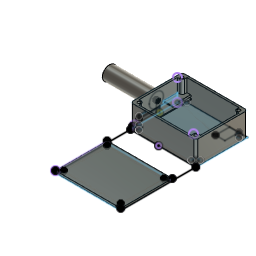
modelo para la plaqueta del nivel v13 (Autodesk Fusion 360 design; units mm, degrees)
Autodesk Fusion 360 part; units mm, degrees
sketch "Boceto1" plane through (0, 0, 0) normal (0, 0, 1) x (1, 0, 0)
  line L0 (39.56, 0) -> (39.56, 55)
  line L1 (39.56, 55) -> (-30, 55)
  line L2 (-30, 55) -> (-30, 0)
  line L3 (-30, 0) -> (39.56, 0)
  dimension "d136" = 55
  dimension "d137" = 69.56
  constraint vertical L0
  constraint horizontal L1
  constraint perpendicular L1 L2
  constraint parallel L1 L3
  constraint coincident origin L3
  measures "d136" distance of L1.end L2.end
  measures "d137" distance of L0.end L1.end
extrude "Extruir1" add sketch "Boceto1" along normal blind 25 makes body 1
shell "Vaciado1" thickness 2 removed faces 1 at (16.3733, 18.3333, 25) on bodies 1
sketch "Boceto2" plane through (0, 0, 0) normal (0, 0, 1) x (1, 0, 0)
  line L0 (-30, -25) -> (39.56, -25)
  line L1 (39.56, -25) -> (39.56, -80)
  line L2 (39.56, -80) -> (-30, -80)
  line L3 (-30, -25) -> (-30, -80)
  line L4 (-30, 0) -> (-30, -25)
  line L5 (39.56, 0) -> (39.56, -25)
  point P0 (-30, 0)
  point P1 (39.56, 0)
  constraint horizontal L0
  constraint vertical L1
  constraint horizontal L2
  constraint perpendicular L2 L3
  constraint coincident P0 L4.start
  constraint perpendicular L0 L4
  constraint coincident P1 L5.start
  constraint perpendicular L0 L5
extrude "Extruir2" add sketch "Boceto2" along normal blind 2 separate body makes body 2
sketch "Boceto7" plane through (0, 0, 2) normal (0, 0, 1) x (-1, 0, 0)
  line L0 (28, -2) -> (-37.56, -2)
  line L1 (-37.56, -2) -> (-37.56, -53)
  line L2 (-37.56, -53) -> (28, -53)
  line L3 (28, -53) -> (28, -2)
  circle A0 centre (25.5, -50.5) radius 2.5
  circle A1 centre (25.5, -4.5) radius 2.5
  circle A2 centre (-35.06, -4.5) radius 2.5
  circle A3 centre (-35.06, -50.5) radius 2.5
  line L4 (23, -50.5) -> (23, -53)
  line L5 (28, -47.9255) -> (25.4266, -48.0011)
  line L6 (25.5, -7) -> (28, -7)
  line L7 (23, -4.5) -> (23, -2)
  line L8 (-32.56, -4.5) -> (-32.56, -2)
  line L9 (-35.06, -7) -> (-37.56, -7)
  line L10 (-34.9754, -48.0014) -> (-37.56, -47.9139)
  line L11 (-32.5302, -53) -> (-32.5602, -50.4704)
  dimension "d26" = 5
  dimension "d27" = 5
  dimension "d28" = 5
  dimension "d29" = 5
  constraint tangent L2 A0
  constraint tangent L3 A0
  constraint tangent L0 A1
  constraint tangent L3 A1
  constraint tangent L1 A3
  constraint tangent L1 A2
  constraint tangent L2 A3
  constraint tangent L0 A2
  constraint coincident A0 L4.start
  constraint coincident L2 L4.end
  constraint tangent A0 L4
  constraint coincident A0 L5.end
  constraint coincident L3 L5.start
  constraint tangent A0 L5
  constraint coincident A1 L6.start
  constraint coincident L3 L6.end
  constraint tangent A1 L6
  constraint coincident A1 L7.start
  constraint coincident L0 L7.end
  constraint tangent A1 L7
  constraint coincident A2 L8.start
  constraint coincident L0 L8.end
  constraint perpendicular L0 L8
  constraint coincident A2 L9.start
  constraint coincident L1 L9.end
  constraint tangent A2 L9
  constraint coincident A3 L10.start
  constraint coincident L1 L10.end
  constraint tangent A3 L10
  constraint coincident A3 L11.end
  constraint coincident L2 L11.start
  constraint tangent A3 L11
  measures "d26" diameter of A0
  measures "d27" diameter of A1
  measures "d28" diameter of A2
  measures "d29" diameter of A3
extrude "Extruir4" add sketch "Boceto7" along normal blind 23 separate body contours A1 | A2 | A0 | A3 L11 makes body 3 at (-27.9876, 50.2511, 17.3333) makes body 4 at (32.5631, 50.6246, 9.6667) makes body 5 at (-27.9969, 4.6246, 9.6667) makes body 6 at (35.7371, 6.9066, 17.3333)
extrude "Extruir5" add sketch "Boceto7" along normal blind 23 contours L0 A1 L7 | L0 A2 L8 | L0 L3 A1 | L0 L1 A2 | L3 A1 L6 | L1 A2 L9 | L3 A0 L5 | L1 A3 L10 | L2 L3 A0 | L1 L2 A3 | L2 A0 L4 | L2 A3 L11 bodies 1 3 4 5 6
sketch "Boceto8" plane through (0, 0, 25) normal (0, 0, 1) x (-1, 0, 0)
  line L0 (30, 0) -> (-39.56, 0)
  line L1 (-39.56, 0) -> (-39.56, -55)
  line L2 (-39.56, -55) -> (30, -55)
  line L3 (30, -55) -> (30, 0)
  arc A0 (25.4266, -48.0011) -> (23, -50.5) centre (25.5, -50.5) ccw
  line L4 (23, -50.5) -> (23, -53)
  line L5 (23, -53) -> (-32.5302, -53)
  line L6 (-32.5302, -53) -> (-32.5602, -50.4704)
  arc A1 (-32.5602, -50.4704) -> (-34.9754, -48.0014) centre (-35.06, -50.5) ccw
  line L7 (-34.9754, -48.0014) -> (-37.56, -47.9139)
  line L8 (-37.56, -47.9139) -> (-37.56, -7)
  line L9 (-37.56, -7) -> (-35.06, -7)
  arc A2 (-35.06, -7) -> (-32.56, -4.5) centre (-35.06, -4.5) ccw
  line L10 (-32.56, -4.5) -> (-32.56, -2)
  line L11 (-32.56, -2) -> (23, -2)
  line L12 (23, -2) -> (23, -4.5)
  arc A3 (23, -4.5) -> (25.5, -7) centre (25.5, -4.5) ccw
  line L13 (25.5, -7) -> (28, -7)
  line L14 (28, -7) -> (28, -47.9255)
  line L15 (28, -47.9255) -> (25.4266, -48.0011)
chamfer "Chaflán4" distance 2 angle 45 1 edges at (39.56, 0, 12.5) on bodies 1
chamfer "Chaflán4" distance 2 angle 45 3 edges at (-30, 0, 12.5) (39.56, 55, 12.5) (-30, 55, 12.5) on bodies 1
chamfer "Chaflán5" distance 2 angle 45 4 edges at (-30, -80, 1) (39.56, -80, 1) (-30, -25, 1) (39.56, -25, 1) on bodies 2
hole "Agujero1" at (-25.5, 50.5, 25) direction (0, 0, -1) diameter 3 depth 20 tip angle 180 bodies 1
hole "Agujero2" at (-25.5, 4.5, 25) direction (0, 0, -1) diameter 3 depth 20 tip angle 180 bodies 1
hole "Agujero7" at (35.06, 4.5, 25) direction (0, 0, -1) diameter 3 depth 20 tip angle 180 bodies 1
hole "Agujero8" at (35.06, 50.5, 25) direction (0, 0, -1) diameter 3 depth 20 tip angle 180 bodies 1
sketch "Boceto9" plane through (0, 0, 2) normal (0, 0, 1) x (-1, 0, 0)
  line L0 (-39.56, 27) -> (-37.56, 25)
  line L1 (-37.56, 25) -> (28, 25)
  line L2 (28, 25) -> (30, 27)
  line L3 (30, 27) -> (30, 78)
  line L4 (30, 78) -> (28, 80)
  line L5 (28, 80) -> (-37.56, 80)
  line L6 (-37.56, 80) -> (-39.56, 78)
  line L7 (-39.56, 78) -> (-39.56, 27)
  circle A0 centre (25.5, 75.5) radius 1.5
  line L8 (30, 25) -> (30, 80)
  circle A1 centre (25.5, 29.5) radius 1.5
  circle A2 centre (-35.06, 75.5) radius 1.5
  circle A3 centre (-35.06, 29.5) radius 1.5
  line L9 (30, 25) -> (25.5, 25)
  line L10 (25.5, 25) -> (25.5, 29.5)
  line L11 (30, 80) -> (25.5, 80)
  line L12 (25.5, 80) -> (25.5, 75.5)
  line L13 (-39.56, 80) -> (-35.06, 80)
  line L14 (-35.06, 80) -> (-35.06, 75.5)
  line L15 (-39.56, 25) -> (-39.56, 29.5)
  line L16 (-39.56, 29.5) -> (-35.06, 29.5)
  point P0 (30, 80)
  point P1 (-39.56, 80)
  point P2 (-39.56, 25)
  dimension "d76" = 3
  dimension "d87" = 3
  dimension "d93" = 3
  dimension "d94" = 3
  dimension "d140" = 4.5
  dimension "d141" = 4.5
  dimension "d142" = 4.5
  dimension "d143" = 4.5
  dimension "d144" = 4.5
  dimension "d145" = 4.5
  dimension "d146" = 4.5
  dimension "d147" = 4.5
  constraint coincident L8.start L9.start
  constraint perpendicular L8 L9
  constraint perpendicular L1 L10
  constraint coincident A1.centre L10.end
  constraint coincident P0 L8.end
  constraint perpendicular L8 L11
  constraint perpendicular L11 L12
  constraint coincident A0.centre L12.end
  constraint coincident P1 L13.start
  constraint parallel L5 L13
  constraint perpendicular L5 L14
  constraint coincident A2.centre L14.end
  constraint coincident P2 L15.start
  constraint parallel L7 L15
  constraint perpendicular L7 L16
  constraint coincident A3.centre L16.end
  measures "d76" diameter of A0
  measures "d87" diameter of A1
  measures "d93" diameter of A2
  measures "d94" diameter of A3
  measures "d140" distance of L8.start L9.end
  measures "d141" distance of L9.end A1.centre
  measures "d142" distance of P0 L11.end
  measures "d143" distance of L11.end A0.centre
  measures "d144" distance of P1 L13.end
  measures "d145" distance of L13.end A2.centre
  measures "d146" distance of P2 L15.end
  measures "d147" distance of L15.end A3.centre
sketch "Boceto11" plane through (-30, 0, 0) normal (-1, 0, 0) x (0, -1, 0)
  line L0 (-53, 25) -> (-53, 0)
  line L1 (-53, 0) -> (-2, 0)
  line L2 (-2, 0) -> (-2, 25)
  line L3 (-2, 25) -> (-53, 25)
  line L4 (-4.5, 2) -> (-2, 2)
  circle A0 centre (-27.5, 13.5) radius 7.5
  line L5 (-27.5, 2) -> (-27.5, 13.5)
  line L6 (-2, 2) -> (-27.5, 2)
  dimension "d125" = 15
  dimension "d138" = 11.5
  dimension "d210" = 25.5
  constraint perpendicular L3 L5
  constraint coincident A0.centre L5.end
  constraint coincident L4.end L6.start
  constraint perpendicular L2 L6
  measures "d125" diameter of A0
  measures "d138" distance of A0.centre L5.start
  measures "d210" distance of L4.end L5.start
hole "Agujero11" at (-25.5, -29.5, 2) at (35.06, -29.5, 2) at (35.06, -75.5, 2) at (-25.5, -75.5, 2) direction (0, 0, -1) diameter 3 depth 3.5 tip angle 180 bodies 2
fillet "Empalme10" radius 1 4 edges at (-26.8985, -28.9576, 2) (33.6615, -28.9576, 2) (33.6615, -74.9576, 2) (-26.8985, -74.9576, 2) on bodies 2
sketch "Boceto13" plane through (-28, 0, 0) normal (1, 0, 0) x (0, 1, 0)
  line L0 (7, 25) -> (7, 2)
  line L1 (7, 2) -> (47.9255, 2)
  line L2 (47.9255, 25) -> (7, 25)
  line L3 (29, 2) -> (29, 7)
  line L4 (29, 7) -> (29, 8)
  line L5 (29, 8) -> (47.9139, 8)
  line L6 (29, 7) -> (47.9139, 7)
  line L7 (29, 7) -> (7, 7)
  line L8 (29, 8) -> (7, 8)
  line L9 (14, 10) -> (7, 10)
  line L10 (47.9139, 8) -> (47.9139, 7)
  line L11 (7, 7) -> (7, 8)
  line L12 (7, 10) -> (14, 10)
  line L13 (7, 8) -> (7, 10)
  line L14 (7, 10) -> (7, 11)
  line L15 (7, 11) -> (14, 11)
  line L16 (14, 11) -> (14, 10)
  line L17 (14, 10) -> (7, 10)
  line L18 (7, 10) -> (7, 11)
  line L19 (47.9139, 8) -> (47.9139, 10)
  line L20 (47.9139, 10) -> (47.9139, 11)
  line L21 (47.9139, 11) -> (32.9139, 11)
  line L22 (32.9139, 11) -> (32.9139, 10)
  line L23 (32.9139, 10) -> (47.9139, 10)
  line L24 (47.9139, 10) -> (47.9139, 11)
  point P0 (29, 2)
  dimension "d163" = 5
  dimension "d164" = 1
  dimension "d193" = 2
  dimension "d194" = 1
  dimension "d195" = 7
  dimension "d196" = 1
  dimension "d197" = 2
  dimension "d198" = 1
  dimension "d199" = 15
  dimension "d200" = 1
  constraint coincident P0 L3.start
  constraint perpendicular L1 L3
  constraint parallel L3 L4
  constraint perpendicular L0 L7
  constraint perpendicular L0 L8
  constraint perpendicular L0 L9
  constraint coincident L0 L9.end
  constraint coincident L0 L8.end
  constraint coincident L0 L7.end
  constraint perpendicular L8 L13
  constraint parallel L0 L14
  constraint horizontal L15
  constraint vertical L16
  constraint horizontal L17
  constraint vertical L18
  constraint perpendicular L5 L19
  constraint horizontal L21
  constraint vertical L22
  constraint horizontal L23
  constraint vertical L24
  measures "d163" distance of P0 L3.end
  measures "d164" distance of L3.end L4.end
  measures "d193" distance of L8.end L9.end
  measures "d194" distance of L9.end L14.end
  measures "d195" distance of L14.end L15.end
  measures "d196" distance of L14.end L9.end
  measures "d197" distance of L5.end L19.end
  measures "d198" distance of L19.end L20.end
  measures "d199" distance of L20.end L21.end
  measures "d200" distance of L20.end L19.end
extrude "Extruir13" add sketch "Boceto13" along normal blind 10 contours L0 L4 L7 L8 L11 bodies 1
extrude "Extruir14" add sketch "Boceto13" along normal blind 10 contours L4 L5 L6 L10 bodies 1
sketch "Boceto15" plane through (0, 0, 2) normal (0, 0, 1) x (-1, 0, 0)
  line L0 (23, -4.5) -> (23, -2)
  line L1 (23, -2) -> (-32.56, -2)
  line L2 (-32.56, -2) -> (-32.56, -4.5)
  arc A0 (-35.06, -7) -> (-32.56, -4.5) centre (-35.06, -4.5) ccw
  line L3 (-35.06, -7) -> (-37.56, -7)
  line L4 (-37.56, -7) -> (-37.56, -47.9139)
  line L5 (-37.56, -47.9139) -> (-34.9754, -48.0014)
  arc A1 (-32.5602, -50.4704) -> (-34.9754, -48.0014) centre (-35.06, -50.5) ccw
  line L6 (-32.5602, -50.4704) -> (-32.5302, -53)
  line L7 (-32.5302, -53) -> (23, -53)
  line L8 (23, -53) -> (23, -50.5)
  arc A2 (25.4266, -48.0011) -> (23, -50.5) centre (25.5, -50.5) ccw
  line L9 (25.4266, -48.0011) -> (28, -47.9255)
  line L10 (28, -47.9255) -> (28, -7)
  line L11 (28, -7) -> (25.5, -7)
  arc A3 (23, -4.5) -> (25.5, -7) centre (25.5, -4.5) ccw
  circle A4 centre (-22.5302, -38) radius 1.5
  circle A5 centre (-22.5302, -38) radius 2.5
  line L12 (-32.5302, -53) -> (-22.5302, -53)
  line L13 (-22.5302, -53) -> (-22.5302, -38)
  line L14 (-22.5302, -38) -> (-32.5302, -38)
  line L15 (-32.5302, -38) -> (-32.5302, -53)
  dimension "d181" = 3
  dimension "d182" = 5
  dimension "d189" = 10
  dimension "d190" = 15
  constraint concentric A4 A5
  constraint horizontal L12
  constraint vertical L13
  constraint horizontal L14
  constraint vertical L15
  constraint coincident L6.end L7.start
  constraint coincident A4.centre A5.centre
  measures "d181" diameter of A4
  measures "d182" diameter of A5
  measures "d189" distance of L6.end L12.end
  measures "d190" distance of L6.end L14.end
extrude "Extruir15" add sketch "Boceto15" along normal blind 5 contours A4 A5 L13 L14 picked at (-24.645, -37.5556) bodies 1
extrude "Extruir16" add sketch "Boceto15" along normal blind 5 contours A4 A5 L13 L14 picked at (-24.6884, -38.1186) bodies 1
extrude "Extruir17" add sketch "Boceto13" along normal blind 10 contours L0 L9 L12 L14 L15 L16 L17 L18 bodies 1
extrude "Extruir18" add sketch "Boceto13" along normal blind 10 contours L20 L21 L22 L23 L24 bodies 1
chamfer "Chaflán9" distance 1 angle 45 2 edges at (-18, 10.5, 11) (-18, 40.4139, 11) on bodies 1
move_face "CarasDesfase1" offset 5 1 faces at (-23, 7, 7.6667) on bodies 1
move_face "CarasDesfase2" offset 5 1 faces at (-20.8333, 7, 10.3333) on bodies 1
move_face "CarasDesfase3" offset 6 1 faces at (-21.6666, 47.9139, 10.3333) on bodies 1
move_face "CarasDesfase4" offset 6 1 faces at (-24.6667, 47.9139, 7.6667) on bodies 1
extrude "Extruir21" add sketch "Boceto11" along normal blind 50 contours A0 bodies 1
hole "Agujero13" at (-80, 27.5, 13.5) direction (1, 0, 0) diameter 11 depth 50 tip angle 180 bodies 1
hole "Agujero16" at (-30, 27.5, 13.5) direction (1, 0, 0) diameter 5 depth 4 tip angle 180 bodies 1
fillet "Empalme11" radius 1 1 edges at (-30, 34.4925, 16.2121) on bodies 1
named bodies: "Cuerpo", "Tapa"
